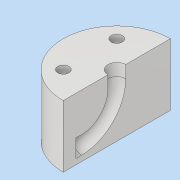
# Autodesk Inventor part: Side1Attachment
Saved by Autodesk Inventor 2017 (Build 210142000, 142)
## iProperties
Created: 2016-11-03
Part Number: Side1Attachment
Material: ABS Plastic
Document SubType Name: Modeling
Designer: techn
Density: 1.06 g/cm^3
Appearance: Smooth - White
Author: techn
Autodesk Inventor part; units mm, degrees
ref_plane "YZ Plane" through (0, 0, 0) normal (1, 0, 0) x (0, 1, 0)
ref_plane "XZ Plane" through (0, 0, 0) normal (0, 1, 0) x (-1, 0, 0)
ref_plane "XY Plane" through (0, 0, 0) normal (0, 0, 1) x (1, 0, 0)
sketch "Sketch1" plane through (0, 0, 0) normal (0, 1, 0) x (-1, 0, 0)
  circle A0 centre (0, 0) radius 12.065
  line L0 (0, 0) -> (6.0168, -6.0168)
  line L1 (0, 0) -> (8.509, 0) construction
  circle A1 centre (6.0168, -6.0168) radius 1.27
  circle A2 centre (6.0168, 6.0168) radius 1.27
  circle A3 centre (-6.0168, 6.0168) radius 1.27
  circle A4 centre (-6.0168, -6.0168) radius 1.27
  dimension "d0" = 24.13
  dimension "d1" = 45
  dimension "d2" = 8.509
  dimension "d3" = 2.54
  dimension "d6" = 360
  constraints: 5 centre point, 4 end point, 2 coincident, 1 equal length, 1 horizontal, 9 other
  measures "d0" diameter of A0
  measures "d1" angle of L0 L1
  measures "d2" distance of L0.start L0.end
  measures "d3" diameter of A1
extrude "Extrusion1" add sketch "Sketch1" along normal blind 13.97
sketch "Sketch2" plane through (0, 0, 0) normal (1, 0, 0) x (0, 1, 0)
  line L0 (13.97, -12.065) -> (13.97, 12.065) projected
  line L1 (13.97, 0) -> (11.2075, 0)
  line L2 (11.2075, 0) -> (3.27, 0)
  line L3 (3.27, 0) -> (3.27, 7.9375)
  line L4 (3.27, 7.9375) -> (3.27, 9.2075)
  line L5 (0, 12.065) -> (0, -12.065) projected
  arc A0 (3.27, 7.9375) -> (11.2075, 0) centre (11.2075, 7.9375) ccw
  point P0 (0, 0)
  dimension "d15" = 7.9375
  dimension "d16" = 7.9375
  dimension "d17" = 1.27
  dimension "d18" = 3.27
  constraints: 8 end point, 2 horizontal, 2 point on circle, 1 centre point, 1 midpoint, 1 parallel, 1 perpendicular, 1 tangent
  measures "d15" distance of L1.end L2.end
  measures "d16" distance of L2.end L3.end
  measures "d17" distance of L3.end L4.end
  measures "d18" distance between parallel lines of L5 L4
sketch "Sketch3" plane through (0, 13.97, 0) normal (0, 1, 0) x (1, 0, 0)
  circle A0 centre (0, 0) radius 2
  dimension "d14" = 4
  constraints: 1 centre point, 1 coincident
  measures "d14" diameter of A0
sweep "Sweep1" cut profiles "Sketch3" path "Sketch2" path curves L1 A0 L4
sketch "Sketch4" plane through (0, 0, 0) normal (1, 0, 0) x (0, 1, 0)
  line L0 (21.6749, -17.4359) -> (-6.3985, -17.4359)
  line L1 (-6.3985, -17.4359) -> (-6.3985, 17.036)
  line L2 (-6.3985, 17.036) -> (21.6749, 17.036)
  line L3 (21.6749, 17.036) -> (21.6749, -17.4359)
  point P0 (0, 0)
  constraints: 8 end point, 2 parallel, 1 horizontal, 1 perpendicular
extrude "Extrusion2" cut sketch "Sketch4" along normal through all
body "Solid1"
